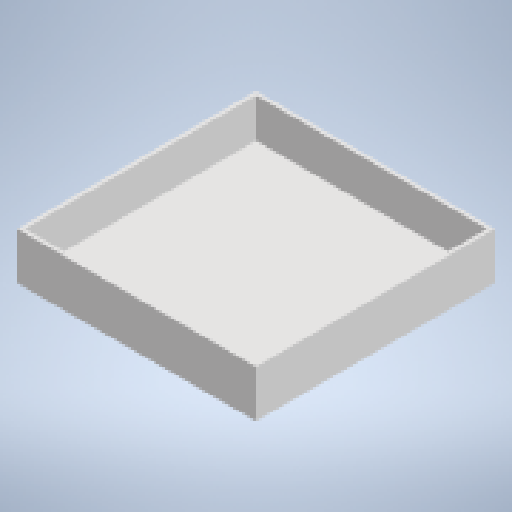
# Autodesk Inventor part: reservatorio
Saved by Autodesk Inventor 2025.1 (Build 291241000, 241)
## iProperties
Created: 2024-11-12
Part Number: reservatorio
Material: Genérico
Document SubType Name: Modeling
Designer: pedro
Density: 1 g/cm^3
Appearance: Padrão
Author: pedro
Autodesk Inventor part; units mm, degrees
ref_plane "YZ Plane" through (0, 0, 0) normal (1, 0, 0) x (0, 1, 0)
ref_plane "XZ Plane" through (0, 0, 0) normal (0, 1, 0) x (-1, 0, 0)
ref_plane "XY Plane" through (0, 0, 0) normal (0, 0, 1) x (1, 0, 0)
sketch "Esboço1" plane through (0, 0, 0) normal (0, 1, 0) x (-1, 0, 0)
  line L0 (152.5, 152.5) -> (-152.5, 152.5)
  line L1 (-152.5, 152.5) -> (-152.5, -152.5)
  line L2 (-152.5, -152.5) -> (152.5, -152.5)
  line L3 (152.5, -152.5) -> (152.5, 152.5)
  point P0 (0, 0)
  dimension "d0" = 305
  dimension "d1" = 305
  dimension "d2" = 152.5
  dimension "d3" = 152.5
  constraints: 8 end point, 2 parallel, 1 horizontal, 1 perpendicular
  measures "d0" distance of L2.end L1.end
  measures "d1" distance of L1.end L0.end
  measures "d2" distance from line of point (0, 0) L0
  measures "d3" distance from line of point (0, 0) L3
extrude "Extrusão1" add sketch "Esboço1" along normal blind 60
sketch "Esboço2" plane through (0, 60, 0) normal (0, 1, 0) x (1, 0, 0)
  line L0 (-147.5, -147.5) -> (147.5, -147.5)
  line L1 (-152.5, -152.5) -> (152.5, -152.5) projected
  line L2 (147.5, -147.5) -> (147.5, 147.5)
  line L3 (-147.5, -147.5) -> (-147.5, 147.5)
  line L4 (-147.5, 147.5) -> (147.5, 147.5)
  line L5 (152.5, 152.5) -> (-152.5, 152.5) projected
  line L6 (152.5, -152.5) -> (152.5, 152.5) projected
  line L7 (-152.5, 152.5) -> (-152.5, -152.5) projected
  point P0 (0, 0)
  dimension "d10" = 5
  dimension "d11" = 5
  dimension "d12" = 5
  dimension "d13" = 5
  constraints: 8 end point, 2 perpendicular, 1 parallel, 1 vertical
  measures "d10" distance between parallel lines of L5 L4
  measures "d11" distance between parallel lines of L6 L2
  measures "d12" distance between parallel lines of L1 L0
  measures "d13" distance between parallel lines of L7 L3
extrude "Extrusão2" cut sketch "Esboço2" against normal blind 50 contours L3 L4 L2 L0
